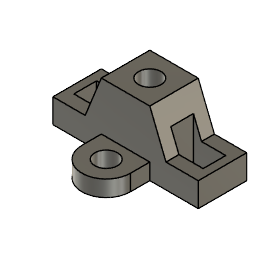
Model_Q5_a (Autodesk Fusion 360 design; units mm, degrees)
part number: 2026-05-25-19-46-14-845
Autodesk Fusion 360 part; units mm, degrees
sketch "Sketch1" plane through (0, 0, 0) normal (0, 1, 0) x (1, 0, 0)
sketch "Sketch2" plane through (0, 0, 0) normal (0, 1, 0) x (1, 0, 0)
  line L0 (0, 0) -> (90, 0)
  line L1 (0, 0) -> (0, -15)
  line L2 (0, -15) -> (90, -15)
  line L3 (90, -15) -> (90, 0)
  line L4 (90, 0) -> (90, -10)
  line L5 (60, -10) -> (30, -10)
  line L6 (90, 0) -> (90, -15)
  line L7 (60, -40) -> (30, -40)
  line L8 (0, -15) -> (20, -15)
  line L9 (20, -15) -> (70, -15)
  line L10 (20, -15) -> (30, -15)
  line L11 (70, -15) -> (60, -15)
  line L12 (20, -15) -> (30, -40)
  line L13 (60, -40) -> (70, -15)
  line L14 (30, -10) -> (30, 0)
  line L15 (60, -10) -> (60, 0)
  dimension "d2" = 90
  dimension "d3" = 15
  dimension "d5" = 10
  dimension "d7" = 20
  dimension "d11" = 50
  dimension "d12" = 10
  dimension "d13" = 10
  dimension "d14" = 20
  constraint coincident L0.start L1.start
  constraint horizontal L0
  constraint perpendicular L0 L1
  constraint perpendicular L1 L2
  constraint perpendicular L0 L4
  constraint perpendicular L1 L5
  constraint perpendicular L2 L6
  constraint perpendicular L6 L7
  constraint perpendicular L1 L8
  constraint parallel L2 L9
  constraint parallel L9 L10
  constraint parallel L9 L11
  constraint coincident L0 L14.end
  constraint perpendicular L0 L14
  constraint coincident L0 L15.end
  constraint perpendicular L0 L15
  measures "d2" distance of L0.start L0.end
  measures "d3" distance of L0.start L1.end
  measures "d5" distance of L0.end L4.end
  measures "d7" distance of L1.end L8.end
  measures "d11" distance of L8.end L9.end
  measures "d12" distance of L8.end L10.end
  measures "d13" distance of L9.end L11.end
  measures "d14" distance of L2.end L9.end
extrude "Extrude1" add sketch "Sketch2" along normal blind 30 contours L0 L1 L2 L3 L4 L5 L6 L8 L9 L10 L11 L14 L15 | L2 L7 L9 L10 L11 L12 L13
sketch "Sketch3" plane through (0, 0, 0) normal (0, 1, 0) x (1, 0, 0)
  line L0 (30, 0) -> (30, -10)
  line L1 (30, -10) -> (60, -10)
  line L2 (60, -10) -> (60, 0)
  line L3 (60, 0) -> (30, 0)
  constraint vertical L0
  constraint perpendicular L0 L1
  constraint perpendicular L1 L2
  constraint perpendicular L0 L3
extrude "Extrude2" add sketch "Sketch3" along normal blind 57
move_body "Move1" bodies 1 to x (-1, 0, 0) y (0, -1, 0) z (0, 0, 1) at (90, 0, 0)
sketch "Sketch4" plane through (0, 0, 0) normal (0, 0, 1) x (1, 0, 0)
  circle A0 through (52, -15, 40) (41.5, -8.9378, 40) (41.5, -21.0622, 40)
  dimension "d20" = 14
extrude "Extrude3" cut sketch "Sketch4" against normal blind 40 contours A0 in plane through (0, 0, 40) normal (0, 0, 1)
delete_face "DeleteFace1" 1 faces at (40, -48, 10)
sketch "Sketch5" plane through (0, 0, 0) normal (0, 0, 1) x (1, 0, 0)
  line L0 (30, -30) -> (30, -42)
  line L1 (30, -42) -> (60, -42)
  line L2 (60, -42) -> (60, -30)
  arc A0 (30, -42) -> (60, -42) centre (45, -42) ccw
  line L3 (30, -30) -> (60, -30)
  dimension "d23" = 12
  constraint vertical L0
  constraint perpendicular L0 L1
  constraint perpendicular L1 L2
  constraint midpoint L1 A0.centre
  constraint perpendicular L2 L3
  measures "d23" distance of L0.start L0.end
extrude "Extrude4" add sketch "Sketch5" along normal blind 10
sketch "Sketch6" plane through (0, 0, 10) normal (0, 0, 1) x (-1, 0, 0)
  arc A0 (-30, 42) -> (-60, 42) centre (-45, 42) ccw
  line L0 (-60, 42) -> (-60, 30)
  line L1 (-60, 30) -> (-30, 30)
  line L2 (-30, 30) -> (-30, 42)
  circle A1 centre (-45, 42) radius 7
  dimension "d26" = 14
  dimension "d27" = 15
  constraint concentric A0 A1
  measures "d26" diameter of A1
  measures "d27" distance of A0.centre L0
extrude "Extrude5" cut sketch "Sketch6" against normal blind 10 contours A1
sketch "Sketch7" plane through (0, 0, 15) normal (0, 0, 1) x (-1, 0, 0)
  line L0 (-90, 0) -> (-70, 0)
  line L1 (-70, 0) -> (-70, 30)
  line L2 (-70, 30) -> (-90, 30)
  line L3 (-90, 30) -> (-90, 0)
  line L4 (-85, 8, 17) -> (-65, 8, 17)
  line L5 (-65, 8, 17) -> (-65, 22, 17)
  line L6 (-65, 22, 17) -> (-85, 22, 17)
  line L7 (-85, 22, 17) -> (-85, 8, 17)
  line L8 (-65, 22, 17) -> (-65, 8, 17)
  line L9 (-65, 8, 17) -> (-85, 8, 17)
extrude "Extrude6" cut sketch "Sketch7" against normal blind 32 contours L4 L5 L6 L7 L8 L9 in plane through (0, 0, 32) normal (0, 0, 1)
sketch "Sketch8" plane through (0, 0, 15) normal (0, 0, 1) x (-1, 0, 0)
  line L0 (-20, 0) -> (0, 0)
  line L1 (0, 0) -> (0, 30)
  line L2 (0, 30) -> (-20, 30)
  line L3 (-20, 30) -> (-20, 0)
  line L4 (-5, 8, 17) -> (-5, 22, 17)
  line L5 (-5, 22, 17) -> (-25, 22, 17)
  line L6 (-25, 22, 17) -> (-25, 8, 17)
  line L7 (-25, 8, 17) -> (-5, 8, 17)
extrude "Extrude7" cut sketch "Sketch8" against normal blind 32 contours L4 L5 L6 L7 in plane through (0, 0, 32) normal (0, 0, 1)
